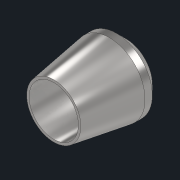
# Autodesk Inventor part: rod330_end_cap
Saved by Autodesk Inventor 2022 (Build 260153000, 153)
## iProperties
Created: 2024-03-31
Part Number: rod330_end_cap
Material: ステンレス鋼
Document SubType Name: Modeling
Designer: gisen
Mass: 58.7818 g
Surface Area: 47.3431 cm^2
Volume: 7.34772 cm^3
Density: 8 g/cm^3
Appearance: 半つや出し
Author: gisen
Autodesk Inventor part; units mm, degrees
ref_plane "YZ Plane" through (0, 0, 0) normal (1, 0, 0) x (0, 1, 0)
ref_plane "XZ Plane" through (0, 0, 0) normal (0, 1, 0) x (-1, 0, 0)
ref_plane "XY Plane" through (0, 0, 0) normal (0, 0, 1) x (1, 0, 0)
sketch "スケッチ1" plane through (0, 0, 0) normal (1, 0, 0) x (0, 1, 0)
  line L0 (10.2, 20) -> (10.2, 0)
  line L1 (10.2, 0) -> (9, 0)
  line L2 (9, 0) -> (9, -10)
  line L3 (9, -10) -> (14.8, -10)
  line L4 (0, -16) -> (0, 26) projected
  line L5 (10.2, 20) -> (14.8, 20)
  line L6 (14.8, 20) -> (14.8, -10)
  point P0 (0, 0)
  dimension "d2" = 10
  dimension "d3" = 10.2
  dimension "d12" = 9
  dimension "d14" = 14.8
  dimension "d15" = 20
  constraints: 12 end point, 3 perpendicular, 2 vertical, 1 horizontal, 1 horizontal alignment
  measures "d2" distance of L1.end L2.end
  measures "d3" distance from line of point (0, 0) L0
  measures "d12" distance between parallel lines of L2 L4
  measures "d14" distance from line of L3.end L4
  measures "d15" distance of L0.start L0.end
revolve "回転1" add sketch "スケッチ1" angle 360 about axis through (0, 0, -10) along (0, 0, 1)
thread "ねじ1" size "M18x2" class "6H" standard "ISO Metric profile" full length
chamfer "面取り1" distance 23 distance2 3.6 1 edges at (0, -14.8, 20) measured on face at (1.1909, 14.752, 0)
chamfer "面取り2" distance 4 angle 45 1 edges at (0, -14.8, -10)
